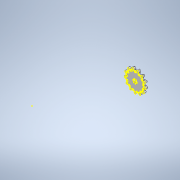
# Autodesk Inventor part: ｍ2歯数13ギア6切削実験甲
Saved by Autodesk Inventor 2020.2 (Build 242310000, 310)
## iProperties
Created: 2020-02-20
Part Number: ｍ2歯数13ギア6切削実験甲
Material: 一般
Document SubType Name: Modeling
Designer: aoyam
Density: 1 g/cm^3
Appearance: 既定
Author: aoyam
Autodesk Inventor part; units mm, degrees
ref_plane "YZ Plane" through (0, 0, 0) normal (1, 0, 0) x (0, 1, 0)
ref_plane "XZ Plane" through (0, 0, 0) normal (0, 1, 0) x (-1, 0, 0)
ref_plane "XY Plane" through (0, 0, 0) normal (0, 0, 1) x (1, 0, 0)
sketch "スケッチ1" plane through (0, 0, 0) normal (0, 0, 1) x (1, 0, 0)
  arc A0 (142.3096, 112.4021) -> (142.2446, 112.1427) centre (143.6618, 111.9254) ccw
  arc A1 (142.6961, 113.2166) -> (142.3096, 112.4021) centre (146.0761, 111.114) ccw
  arc A2 (143.9239, 114.698) -> (142.6961, 113.2166) centre (148.6702, 109.5145) ccw
  arc A3 (139.6615, 112.1427) -> (139.5965, 112.4021) centre (138.2443, 111.9254) ccw
  arc A4 (139.5965, 112.4021) -> (139.21, 113.2166) centre (135.83, 111.114) ccw
  arc A5 (139.21, 113.2166) -> (137.9821, 114.698) centre (133.2359, 109.5145) ccw
  arc A6 (142.0632, 110.4363) -> (139.8429, 110.4363) centre (140.953, 99.9952) ccw
  arc A7 (137.9821, 114.698) -> (136.7509, 114.3945) centre (140.953, 99.9952) ccw
  line L0 (142.0632, 110.4363) -> (142.2446, 112.1427)
  line L1 (139.8429, 110.4363) -> (139.6615, 112.1427)
  arc A8 (136.3884, 111.6113) -> (136.4514, 111.3515) centre (137.8072, 111.8177) ccw
  line L2 (137.0838, 109.7563) -> (136.4514, 111.3515)
  arc A9 (136.3521, 112.5122) -> (136.3884, 111.6113) centre (140.3221, 112.2212) ccw
  arc A10 (136.7509, 114.3945) -> (136.3521, 112.5122) centre (143.3624, 112.0105) ccw
  arc A11 (137.0838, 109.7563) -> (135.1178, 108.7244) centre (140.953, 99.9952) ccw
  line L3 (135.1178, 108.7244) -> (134.1642, 110.1511)
  arc A12 (134.1642, 110.1511) -> (133.9861, 110.3505) centre (133.0103, 109.3001) ccw
  arc A13 (133.9861, 110.3505) -> (133.2653, 110.8922) centre (131.2496, 107.4596) ccw
  arc A14 (133.2653, 110.8922) -> (131.4897, 111.6333) centre (129.696, 104.8378) ccw
  arc A15 (131.4897, 111.6333) -> (130.5405, 110.7923) centre (140.953, 99.9952) ccw
  arc A16 (131.513, 108.1595) -> (131.6895, 107.9587) centre (132.6734, 109.0016) ccw
  line L4 (132.9908, 106.84) -> (131.6895, 107.9587)
  arc A17 (131.0621, 108.9403) -> (131.513, 108.1595) centre (134.7127, 110.5276) ccw
  arc A18 (130.5405, 110.7923) -> (131.0621, 108.9403) centre (137.5026, 111.7539) ccw
  arc A19 (132.9908, 106.84) -> (131.7295, 105.0128) centre (140.953, 99.9952) ccw
  line L5 (131.7295, 105.0128) -> (130.2221, 105.8328)
  arc A20 (130.2221, 105.8328) -> (129.9718, 105.9267) centre (129.5959, 104.5431) ccw
  arc A21 (129.9718, 105.9267) -> (129.0818, 106.0713) centre (128.8922, 102.0952) ccw
  arc A22 (129.0818, 106.0713) -> (127.1652, 105.9023) centre (128.7349, 99.0517) ccw
  arc A23 (127.1652, 105.9023) -> (126.7155, 104.7166) centre (140.953, 99.9952) ccw
  arc A24 (128.8001, 102.8373) -> (129.0498, 102.7416) centre (129.4363, 104.1222) ccw
  line L6 (130.7218, 102.3558) -> (129.0498, 102.7416)
  arc A25 (128.0381, 103.3192) -> (128.8001, 102.8373) centre (130.5328, 106.4211) ccw
  arc A26 (126.7155, 104.7166) -> (128.0381, 103.3192) centre (132.4333, 108.8035) ccw
  arc A27 (130.7218, 102.3558) -> (130.4542, 100.1517) centre (140.953, 99.9952) ccw
  line L7 (130.4542, 100.1517) -> (128.7384, 100.1772)
  arc A28 (128.7384, 100.1772) -> (128.4731, 100.144) centre (128.7832, 98.7442) ccw
  arc A29 (128.4731, 100.144) -> (127.6179, 99.8585) centre (129.2978, 96.2497) ccw
  arc A30 (127.6179, 99.8585) -> (125.9993, 98.8182) centre (130.5729, 93.4817) ccw
  arc A31 (125.9993, 98.8182) -> (126.1521, 97.5593) centre (140.953, 99.9952) ccw
  arc A32 (128.8714, 96.864) -> (129.1369, 96.8952) centre (128.8375, 98.2974) ccw
  line L8 (130.7967, 97.3307) -> (129.1369, 96.8952)
  arc A33 (127.9727, 96.9365) -> (128.8714, 96.864) centre (128.7401, 100.8426) ccw
  arc A34 (126.1521, 97.5593) -> (127.9727, 96.9365) centre (129.3158, 103.8352) ccw
  arc A35 (130.7967, 97.3307) -> (131.5841, 95.2547) centre (140.953, 99.9952) ccw
  line L9 (131.5841, 95.2547) -> (130.0529, 94.48)
  arc A36 (130.0529, 94.48) -> (129.8334, 94.3272) centre (130.7586, 93.2319) ccw
  arc A37 (129.8334, 94.3272) -> (129.2089, 93.677) centre (132.3734, 91.2622) ccw
  arc A38 (129.2089, 93.677) -> (128.2591, 92.0036) centre (134.7888, 89.4039) ccw
  arc A39 (128.2591, 92.0036) -> (128.9795, 90.96) centre (140.953, 99.9952) ccw
  arc A40 (131.7104, 91.608) -> (131.931, 91.7591) centre (131.0143, 92.8615) ccw
  line L10 (133.1983, 92.916) -> (131.931, 91.7591)
  arc A41 (130.8809, 91.2546) -> (131.7104, 91.608) centre (129.7452, 95.0699) ccw
  arc A42 (128.9795, 90.96) -> (130.8809, 91.2546) centre (128.8642, 97.9872) ccw
  arc A43 (133.1983, 92.916) -> (134.8602, 91.4437) centre (140.953, 99.9952) ccw
  line L11 (134.8602, 91.4437) -> (133.8645, 90.0461)
  arc A44 (133.8645, 90.0461) -> (133.7411, 89.8089) centre (135.0693, 89.269) ccw
  arc A45 (133.7411, 89.8089) -> (133.4903, 88.9429) centre (137.4146, 88.2754) ccw
  arc A46 (133.4903, 88.9429) -> (133.427, 87.0199) centre (140.4169, 87.7524) ccw
  arc A47 (133.427, 87.0199) -> (134.5498, 86.4305) centre (140.953, 99.9952) ccw
  arc A48 (136.6667, 88.2735) -> (136.7919, 88.5097) centre (135.4679, 89.0598) ccw
  line L12 (137.3764, 90.1231) -> (136.7919, 88.5097)
  arc A49 (136.0966, 87.575) -> (136.6667, 88.2735) centre (133.3179, 90.4255) ccw
  arc A50 (134.5498, 86.4305) -> (136.0966, 87.575) centre (131.182, 92.5993) ccw
  arc A51 (137.3764, 90.1231) -> (139.5322, 89.5917) centre (140.953, 99.9952) ccw
  line L13 (139.5322, 89.5917) -> (139.3, 87.8915)
  arc A52 (139.3, 87.8915) -> (139.301, 87.6242) centre (140.728, 87.7633) ccw
  arc A53 (139.301, 87.6242) -> (139.4813, 86.7408) centre (143.2663, 87.9734) ccw
  arc A54 (139.4813, 86.7408) -> (140.319, 85.0086) centre (146.1678, 88.9056) ccw
  arc A55 (140.319, 85.0086) -> (141.5871, 85.0086) centre (140.953, 99.9952) ccw
  arc A56 (142.6051, 87.6242) -> (142.6061, 87.8915) centre (141.1781, 87.7633) ccw
  line L14 (142.3739, 89.5917) -> (142.6061, 87.8915)
  arc A57 (142.4248, 86.7408) -> (142.6051, 87.6242) centre (138.6397, 87.9734) ccw
  arc A58 (141.5871, 85.0086) -> (142.4248, 86.7408) centre (135.7383, 88.9056) ccw
  arc A59 (142.3739, 89.5917) -> (144.5297, 90.1231) centre (140.953, 99.9952) ccw
  line L15 (144.5297, 90.1231) -> (145.1142, 88.5097)
  arc A60 (145.1142, 88.5097) -> (145.2393, 88.2735) centre (146.4382, 89.0598) ccw
  arc A61 (145.2393, 88.2735) -> (145.8095, 87.575) centre (148.5882, 90.4255) ccw
  arc A62 (145.8095, 87.575) -> (147.3562, 86.4305) centre (150.7241, 92.5993) ccw
  arc A63 (147.3562, 86.4305) -> (148.4791, 87.0199) centre (140.953, 99.9952) ccw
  arc A64 (148.1649, 89.8089) -> (148.0416, 90.0461) centre (146.8367, 89.269) ccw
  line L16 (147.0458, 91.4437) -> (148.0416, 90.0461)
  arc A65 (148.4158, 88.9429) -> (148.1649, 89.8089) centre (144.4915, 88.2754) ccw
  arc A66 (148.4791, 87.0199) -> (148.4158, 88.9429) centre (141.4892, 87.7524) ccw
  arc A67 (147.0458, 91.4437) -> (148.7078, 92.916) centre (140.953, 99.9952) ccw
  line L17 (148.7078, 92.916) -> (149.9751, 91.7591)
  arc A68 (149.9751, 91.7591) -> (150.1957, 91.608) centre (150.8918, 92.8615) ccw
  arc A69 (150.1957, 91.608) -> (151.0252, 91.2546) centre (152.1608, 95.0699) ccw
  arc A70 (151.0252, 91.2546) -> (152.9266, 90.96) centre (153.0419, 97.9872) ccw
  arc A71 (152.9266, 90.96) -> (153.6469, 92.0036) centre (140.953, 99.9952) ccw
  arc A72 (152.0726, 94.3272) -> (151.8532, 94.48) centre (151.1475, 93.2319) ccw
  line L18 (150.322, 95.2547) -> (151.8532, 94.48)
  arc A73 (152.6972, 93.677) -> (152.0726, 94.3272) centre (149.5326, 91.2622) ccw
  arc A74 (153.6469, 92.0036) -> (152.6972, 93.677) centre (147.1172, 89.4039) ccw
  arc A75 (150.322, 95.2547) -> (151.1093, 97.3307) centre (140.953, 99.9952) ccw
  line L19 (151.1093, 97.3307) -> (152.7692, 96.8952)
  arc A76 (152.7692, 96.8952) -> (153.0347, 96.864) centre (153.0686, 98.2974) ccw
  arc A77 (153.0347, 96.864) -> (153.9334, 96.9365) centre (153.166, 100.8426) ccw
  arc A78 (153.9334, 96.9365) -> (155.7539, 97.5593) centre (152.5903, 103.8352) ccw
  arc A79 (155.7539, 97.5593) -> (155.9068, 98.8182) centre (140.953, 99.9952) ccw
  arc A80 (153.433, 100.144) -> (153.1677, 100.1772) centre (153.1228, 98.7442) ccw
  line L20 (151.4519, 100.1517) -> (153.1677, 100.1772)
  arc A81 (154.2882, 99.8585) -> (153.433, 100.144) centre (152.6083, 96.2497) ccw
  arc A82 (155.9068, 98.8182) -> (154.2882, 99.8585) centre (151.3332, 93.4817) ccw
  arc A83 (151.4519, 100.1517) -> (151.1842, 102.3558) centre (140.953, 99.9952) ccw
  line L21 (151.1842, 102.3558) -> (152.8563, 102.7416)
  arc A84 (152.8563, 102.7416) -> (153.1059, 102.8373) centre (152.4698, 104.1222) ccw
  arc A85 (153.1059, 102.8373) -> (153.868, 103.3192) centre (151.3732, 106.4211) ccw
  arc A86 (153.868, 103.3192) -> (155.1906, 104.7166) centre (149.4728, 108.8035) ccw
  arc A87 (155.1906, 104.7166) -> (154.7409, 105.9023) centre (140.953, 99.9952) ccw
  arc A88 (151.9343, 105.9267) -> (151.684, 105.8328) centre (152.3102, 104.5431) ccw
  line L22 (150.1766, 105.0128) -> (151.684, 105.8328)
  arc A89 (152.8242, 106.0713) -> (151.9343, 105.9267) centre (153.0139, 102.0952) ccw
  arc A90 (154.7409, 105.9023) -> (152.8242, 106.0713) centre (153.1711, 99.0517) ccw
  arc A91 (150.1766, 105.0128) -> (148.9153, 106.84) centre (140.953, 99.9952) ccw
  line L23 (148.9153, 106.84) -> (150.2166, 107.9587)
  arc A92 (150.2166, 107.9587) -> (150.3931, 108.1595) centre (149.2327, 109.0016) ccw
  arc A93 (150.3931, 108.1595) -> (150.8439, 108.9403) centre (147.1934, 110.5276) ccw
  arc A94 (150.8439, 108.9403) -> (151.3656, 110.7923) centre (144.4035, 111.7539) ccw
  arc A95 (151.3656, 110.7923) -> (150.4164, 111.6333) centre (140.953, 99.9952) ccw
  arc A96 (147.92, 110.3505) -> (147.7419, 110.1511) centre (148.8958, 109.3001) ccw
  line L24 (146.7883, 108.7244) -> (147.7419, 110.1511)
  arc A97 (148.6407, 110.8922) -> (147.92, 110.3505) centre (150.6565, 107.4596) ccw
  arc A98 (150.4164, 111.6333) -> (148.6407, 110.8922) centre (152.2101, 104.8378) ccw
  arc A99 (146.7883, 108.7244) -> (144.8223, 109.7563) centre (140.953, 99.9952) ccw
  line L25 (144.8223, 109.7563) -> (145.4546, 111.3515)
  arc A100 (145.4546, 111.3515) -> (145.5176, 111.6113) centre (144.0988, 111.8177) ccw
  arc A101 (145.5176, 111.6113) -> (145.554, 112.5122) centre (141.5839, 112.2212) ccw
  arc A102 (145.554, 112.5122) -> (145.1552, 114.3945) centre (138.5437, 112.0105) ccw
  arc A103 (145.1552, 114.3945) -> (143.9239, 114.698) centre (140.953, 99.9952) ccw
  circle A104 centre (140.953, 99.9952) radius 10.5 construction
  circle A105 centre (140.953, 99.9952) radius 15 construction
  line L26 (140.7262, 102.7971) -> (141.8821, 102.6483)
  line L27 (143.2661, 101.5926) -> (143.7152, 100.5172)
  line L28 (143.493, 98.7907) -> (142.7862, 97.8641)
  line L29 (141.1799, 97.1933) -> (140.024, 97.3421)
  line L30 (138.64, 98.3978) -> (138.1909, 99.4732)
  line L31 (138.4131, 101.1996) -> (139.1199, 102.1263)
  arc A106 (140.7262, 102.7971) -> (139.1199, 102.1263) centre (140.1167, 101.998) ccw
  arc A107 (138.4131, 101.1996) -> (138.1909, 99.4732) centre (138.8004, 100.2723) ccw
  arc A108 (138.64, 98.3978) -> (140.024, 97.3421) centre (139.6367, 98.2694) ccw
  arc A109 (141.1799, 97.1933) -> (142.7862, 97.8641) centre (141.7894, 97.9924) ccw
  arc A110 (143.493, 98.7907) -> (143.7152, 100.5172) centre (143.1057, 99.7181) ccw
  arc A111 (143.2661, 101.5926) -> (141.8821, 102.6483) centre (142.2693, 101.7209) ccw
  point P0 (0, 0)
  point P1 (140.953, 116.9952)
  point P2 (133.0527, 115.0479)
  point P3 (126.9623, 109.6523)
  point P4 (124.077, 102.0443)
  point P5 (125.0578, 93.9669)
  point P6 (129.6799, 87.2705)
  point P7 (136.8847, 83.4892)
  point P8 (145.0214, 83.4892)
  point P9 (152.2261, 87.2705)
  point P10 (156.8483, 93.9669)
  point P11 (157.8291, 102.0443)
  point P12 (154.9438, 109.6523)
  point P13 (148.8533, 115.0479)
  point P14 (139.7294, 102.9254)
  point P15 (137.8036, 100.4006)
  point P16 (139.0272, 97.4704)
  point P17 (142.1767, 97.065)
  point P18 (144.1025, 99.5898)
  point P19 (142.8788, 102.52)
  point P20 (145.2393, 88.2735)
  point P21 (145.8095, 87.575)
  point P22 (147.3562, 86.4305)
  point P23 (148.4791, 87.0199)
  point P24 (148.4158, 88.9429)
  point P25 (148.0416, 90.0461)
  point P26 (147.0458, 91.4437)
  point P27 (148.7078, 92.916)
  point P28 (150.1957, 91.608)
  point P29 (151.0252, 91.2546)
  point P30 (152.9266, 90.96)
  point P31 (153.6469, 92.0036)
  point P32 (152.6972, 93.677)
  point P33 (152.0726, 94.3272)
  point P34 (153.0347, 96.864)
  point P35 (153.9334, 96.9365)
  point P36 (155.7539, 97.5593)
  point P37 (155.9068, 98.8182)
  point P38 (154.2882, 99.8585)
  point P39 (153.433, 100.144)
  point P40 (153.1677, 100.1772)
  point P41 (151.4519, 100.1517)
  point P42 (153.1059, 102.8373)
  point P43 (153.868, 103.3192)
  point P44 (155.1906, 104.7166)
  point P45 (154.7409, 105.9023)
  point P46 (152.8242, 106.0713)
  point P47 (151.9343, 105.9267)
  point P48 (150.2166, 107.9587)
  point P49 (150.3931, 108.1595)
  point P50 (151.3656, 110.7923)
  point P51 (150.4164, 111.6333)
  point P52 (148.6407, 110.8922)
  point P53 (147.7419, 110.1511)
  point P54 (145.4546, 111.3515)
  point P55 (145.5176, 111.6113)
  point P56 (145.554, 112.5122)
  point P57 (145.1552, 114.3945)
  point P58 (143.9239, 114.698)
  point P59 (142.6961, 113.2166)
  point P60 (142.2446, 112.1427)
  point P61 (139.6615, 112.1427)
  point P62 (139.5965, 112.4021)
  point P63 (139.21, 113.2166)
  point P64 (136.3884, 111.6113)
  point P65 (137.0838, 109.7563)
  point P66 (135.1178, 108.7244)
  point P67 (133.9861, 110.3505)
  point P68 (133.2653, 110.8922)
  point P69 (131.513, 108.1595)
  point P70 (130.2221, 105.8328)
  point P71 (129.0818, 106.0713)
  point P72 (127.1652, 105.9023)
  point P73 (126.7155, 104.7166)
  point P74 (128.8001, 102.8373)
  point P75 (127.6179, 99.8585)
  point P76 (126.1521, 97.5593)
  point P77 (127.9727, 96.9365)
  point P78 (128.8714, 96.864)
  point P79 (129.8334, 94.3272)
  point P80 (129.2089, 93.677)
  point P81 (128.2591, 92.0036)
  point P82 (128.9795, 90.96)
  point P83 (131.7104, 91.608)
  point P84 (133.1983, 92.916)
  point P85 (133.7411, 89.8089)
  point P86 (133.4903, 88.9429)
  point P87 (134.5498, 86.4305)
  point P88 (136.0966, 87.575)
  point P89 (136.6667, 88.2735)
  point P90 (136.7919, 88.5097)
  point P91 (137.3764, 90.1231)
  point P92 (139.301, 87.6242)
  point P93 (139.4813, 86.7408)
  point P94 (140.319, 85.0086)
  point P95 (142.4248, 86.7408)
  dimension "d4" = 360
  dimension "d10" = 5.5
  dimension "d11" = 2.01
  dimension "d14" = 360
  dimension "d18" = 30
  constraints: 226 point on circle, 112 centre point, 64 end point, 4 coincident, 1 concentric, 537 other
  measures "d10" distance between parallel lines of L30 L27
  measures "d11" diameter of A106
  measures "d18" diameter of A105
extrude "押し出し1" add sketch "スケッチ1" along normal blind 3
sketch "スケッチ2" plane through (0, 0, 3) normal (0, 0, 1) x (1, 0, 0)
  arc A0 (148.4791, 87.0199) -> (148.4158, 88.9429) centre (141.4892, 87.7524) ccw projected
  arc A1 (148.4158, 88.9429) -> (148.1649, 89.8089) centre (144.4915, 88.2754) ccw projected
  arc A2 (148.1649, 89.8089) -> (148.0416, 90.0461) centre (146.8367, 89.269) ccw projected
  line L0 (148.0416, 90.0461) -> (147.0458, 91.4437) projected
  arc A3 (147.0458, 91.4437) -> (148.7078, 92.916) centre (140.953, 99.9952) ccw projected
  line L1 (148.7078, 92.916) -> (149.9751, 91.7591) projected
  arc A4 (149.9751, 91.7591) -> (150.1957, 91.608) centre (150.8918, 92.8615) ccw projected
  arc A5 (150.1957, 91.608) -> (151.0252, 91.2546) centre (152.1608, 95.0699) ccw projected
  arc A6 (151.0252, 91.2546) -> (152.9266, 90.96) centre (153.0419, 97.9872) ccw projected
  arc A7 (152.9266, 90.96) -> (153.6469, 92.0036) centre (140.953, 99.9952) ccw projected
  arc A8 (153.6469, 92.0036) -> (152.6972, 93.677) centre (147.1172, 89.4039) ccw projected
  arc A9 (152.6972, 93.677) -> (152.0726, 94.3272) centre (149.5326, 91.2622) ccw projected
  arc A10 (152.0726, 94.3272) -> (151.8532, 94.48) centre (151.1475, 93.2319) ccw projected
  line L2 (151.8532, 94.48) -> (150.322, 95.2547) projected
  arc A11 (150.322, 95.2547) -> (151.1093, 97.3307) centre (140.953, 99.9952) ccw projected
  line L3 (151.1093, 97.3307) -> (152.7692, 96.8952) projected
  arc A12 (152.7692, 96.8952) -> (153.0347, 96.864) centre (153.0686, 98.2974) ccw projected
  arc A13 (153.0347, 96.864) -> (153.9334, 96.9365) centre (153.166, 100.8426) ccw projected
  arc A14 (153.9334, 96.9365) -> (155.7539, 97.5593) centre (152.5903, 103.8352) ccw projected
  arc A15 (155.7539, 97.5593) -> (155.9068, 98.8182) centre (140.953, 99.9952) ccw projected
  arc A16 (155.9068, 98.8182) -> (154.2882, 99.8585) centre (151.3332, 93.4817) ccw projected
  arc A17 (154.2882, 99.8585) -> (153.433, 100.144) centre (152.6083, 96.2497) ccw projected
  arc A18 (153.433, 100.144) -> (153.1677, 100.1772) centre (153.1228, 98.7442) ccw projected
  line L4 (153.1677, 100.1772) -> (151.4519, 100.1517) projected
  arc A19 (151.4519, 100.1517) -> (151.1842, 102.3558) centre (140.953, 99.9952) ccw projected
  line L5 (151.1842, 102.3558) -> (152.8563, 102.7416) projected
  arc A20 (152.8563, 102.7416) -> (153.1059, 102.8373) centre (152.4698, 104.1222) ccw projected
  arc A21 (153.1059, 102.8373) -> (153.868, 103.3192) centre (151.3732, 106.4211) ccw projected
  arc A22 (153.868, 103.3192) -> (155.1906, 104.7166) centre (149.4728, 108.8035) ccw projected
  arc A23 (155.1906, 104.7166) -> (154.7409, 105.9023) centre (140.953, 99.9952) ccw projected
  arc A24 (154.7409, 105.9023) -> (152.8242, 106.0713) centre (153.1711, 99.0517) ccw projected
  arc A25 (152.8242, 106.0713) -> (151.9343, 105.9267) centre (153.0139, 102.0952) ccw projected
  arc A26 (151.9343, 105.9267) -> (151.684, 105.8328) centre (152.3102, 104.5431) ccw projected
  line L6 (151.684, 105.8328) -> (150.1766, 105.0128) projected
  arc A27 (150.1766, 105.0128) -> (148.9153, 106.84) centre (140.953, 99.9952) ccw projected
  line L7 (148.9153, 106.84) -> (150.2166, 107.9587) projected
  arc A28 (150.2166, 107.9587) -> (150.3931, 108.1595) centre (149.2327, 109.0016) ccw projected
  arc A29 (150.3931, 108.1595) -> (150.8439, 108.9403) centre (147.1934, 110.5276) ccw projected
  arc A30 (150.8439, 108.9403) -> (151.3656, 110.7923) centre (144.4035, 111.7539) ccw projected
  arc A31 (151.3656, 110.7923) -> (150.4164, 111.6333) centre (140.953, 99.9952) ccw projected
  arc A32 (150.4164, 111.6333) -> (148.6407, 110.8922) centre (152.2101, 104.8378) ccw projected
  arc A33 (148.6407, 110.8922) -> (147.92, 110.3505) centre (150.6565, 107.4596) ccw projected
  arc A34 (147.92, 110.3505) -> (147.7419, 110.1511) centre (148.8958, 109.3001) ccw projected
  line L8 (147.7419, 110.1511) -> (146.7883, 108.7244) projected
  arc A35 (146.7883, 108.7244) -> (144.8223, 109.7563) centre (140.953, 99.9952) ccw projected
  line L9 (144.8223, 109.7563) -> (145.4546, 111.3515) projected
  arc A36 (145.4546, 111.3515) -> (145.5176, 111.6113) centre (144.0988, 111.8177) ccw projected
  arc A37 (145.5176, 111.6113) -> (145.554, 112.5122) centre (141.5839, 112.2212) ccw projected
  arc A38 (145.554, 112.5122) -> (145.1552, 114.3945) centre (138.5437, 112.0105) ccw projected
  arc A39 (145.1552, 114.3945) -> (143.9239, 114.698) centre (140.953, 99.9952) ccw projected
  arc A40 (143.9239, 114.698) -> (142.6961, 113.2166) centre (148.6702, 109.5145) ccw projected
  arc A41 (142.6961, 113.2166) -> (142.3096, 112.4021) centre (146.0761, 111.114) ccw projected
  arc A42 (142.3096, 112.4021) -> (142.2446, 112.1427) centre (143.6618, 111.9254) ccw projected
  line L10 (142.2446, 112.1427) -> (142.0632, 110.4363) projected
  arc A43 (142.0632, 110.4363) -> (139.8429, 110.4363) centre (140.953, 99.9952) ccw projected
  line L11 (139.8429, 110.4363) -> (139.6615, 112.1427) projected
  arc A44 (139.6615, 112.1427) -> (139.5965, 112.4021) centre (138.2443, 111.9254) ccw projected
  arc A45 (139.5965, 112.4021) -> (139.21, 113.2166) centre (135.83, 111.114) ccw projected
  arc A46 (139.21, 113.2166) -> (137.9821, 114.698) centre (133.2359, 109.5145) ccw projected
  arc A47 (137.9821, 114.698) -> (136.7509, 114.3945) centre (140.953, 99.9952) ccw projected
  arc A48 (136.7509, 114.3945) -> (136.3521, 112.5122) centre (143.3624, 112.0105) ccw projected
  arc A49 (136.3521, 112.5122) -> (136.3884, 111.6113) centre (140.3221, 112.2212) ccw projected
  arc A50 (136.3884, 111.6113) -> (136.4514, 111.3515) centre (137.8072, 111.8177) ccw projected
  line L12 (136.4514, 111.3515) -> (137.0838, 109.7563) projected
  arc A51 (137.0838, 109.7563) -> (135.1178, 108.7244) centre (140.953, 99.9952) ccw projected
  line L13 (135.1178, 108.7244) -> (134.1642, 110.1511) projected
  arc A52 (134.1642, 110.1511) -> (133.9861, 110.3505) centre (133.0103, 109.3001) ccw projected
  arc A53 (133.9861, 110.3505) -> (133.2653, 110.8922) centre (131.2496, 107.4596) ccw projected
  arc A54 (133.2653, 110.8922) -> (131.4897, 111.6333) centre (129.696, 104.8378) ccw projected
  arc A55 (131.4897, 111.6333) -> (130.5405, 110.7923) centre (140.953, 99.9952) ccw projected
  arc A56 (130.5405, 110.7923) -> (131.0621, 108.9403) centre (137.5026, 111.7539) ccw projected
  arc A57 (131.0621, 108.9403) -> (131.513, 108.1595) centre (134.7127, 110.5276) ccw projected
  arc A58 (131.513, 108.1595) -> (131.6895, 107.9587) centre (132.6734, 109.0016) ccw projected
  line L14 (131.6895, 107.9587) -> (132.9908, 106.84) projected
  arc A59 (132.9908, 106.84) -> (131.7295, 105.0128) centre (140.953, 99.9952) ccw projected
  line L15 (131.7295, 105.0128) -> (130.2221, 105.8328) projected
  arc A60 (130.2221, 105.8328) -> (129.9718, 105.9267) centre (129.5959, 104.5431) ccw projected
  arc A61 (129.9718, 105.9267) -> (129.0818, 106.0713) centre (128.8922, 102.0952) ccw projected
  arc A62 (129.0818, 106.0713) -> (127.1652, 105.9023) centre (128.7349, 99.0517) ccw projected
  arc A63 (127.1652, 105.9023) -> (126.7155, 104.7166) centre (140.953, 99.9952) ccw projected
  arc A64 (126.7155, 104.7166) -> (128.0381, 103.3192) centre (132.4333, 108.8035) ccw projected
  arc A65 (128.0381, 103.3192) -> (128.8001, 102.8373) centre (130.5328, 106.4211) ccw projected
  arc A66 (128.8001, 102.8373) -> (129.0498, 102.7416) centre (129.4363, 104.1222) ccw projected
  line L16 (129.0498, 102.7416) -> (130.7218, 102.3558) projected
  arc A67 (130.7218, 102.3558) -> (130.4542, 100.1517) centre (140.953, 99.9952) ccw projected
  line L17 (130.4542, 100.1517) -> (128.7384, 100.1772) projected
  arc A68 (128.7384, 100.1772) -> (128.4731, 100.144) centre (128.7832, 98.7442) ccw projected
  arc A69 (128.4731, 100.144) -> (127.6179, 99.8585) centre (129.2978, 96.2497) ccw projected
  arc A70 (127.6179, 99.8585) -> (125.9993, 98.8182) centre (130.5729, 93.4817) ccw projected
  arc A71 (125.9993, 98.8182) -> (126.1521, 97.5593) centre (140.953, 99.9952) ccw projected
  arc A72 (126.1521, 97.5593) -> (127.9727, 96.9365) centre (129.3158, 103.8352) ccw projected
  arc A73 (127.9727, 96.9365) -> (128.8714, 96.864) centre (128.7401, 100.8426) ccw projected
  arc A74 (128.8714, 96.864) -> (129.1369, 96.8952) centre (128.8375, 98.2974) ccw projected
  line L18 (129.1369, 96.8952) -> (130.7967, 97.3307) projected
  arc A75 (130.7967, 97.3307) -> (131.5841, 95.2547) centre (140.953, 99.9952) ccw projected
  line L19 (131.5841, 95.2547) -> (130.0529, 94.48) projected
  arc A76 (130.0529, 94.48) -> (129.8334, 94.3272) centre (130.7586, 93.2319) ccw projected
  arc A77 (129.8334, 94.3272) -> (129.2089, 93.677) centre (132.3734, 91.2622) ccw projected
  arc A78 (129.2089, 93.677) -> (128.2591, 92.0036) centre (134.7888, 89.4039) ccw projected
  arc A79 (128.2591, 92.0036) -> (128.9795, 90.96) centre (140.953, 99.9952) ccw projected
  arc A80 (128.9795, 90.96) -> (130.8809, 91.2546) centre (128.8642, 97.9872) ccw projected
  arc A81 (130.8809, 91.2546) -> (131.7104, 91.608) centre (129.7452, 95.0699) ccw projected
  arc A82 (131.7104, 91.608) -> (131.931, 91.7591) centre (131.0143, 92.8615) ccw projected
  line L20 (131.931, 91.7591) -> (133.1983, 92.916) projected
  arc A83 (133.1983, 92.916) -> (134.8602, 91.4437) centre (140.953, 99.9952) ccw projected
  line L21 (134.8602, 91.4437) -> (133.8645, 90.0461) projected
  arc A84 (133.8645, 90.0461) -> (133.7411, 89.8089) centre (135.0693, 89.269) ccw projected
  arc A85 (133.7411, 89.8089) -> (133.4903, 88.9429) centre (137.4146, 88.2754) ccw projected
  arc A86 (133.4903, 88.9429) -> (133.427, 87.0199) centre (140.4169, 87.7524) ccw projected
  arc A87 (133.427, 87.0199) -> (134.5498, 86.4305) centre (140.953, 99.9952) ccw projected
  arc A88 (134.5498, 86.4305) -> (136.0966, 87.575) centre (131.182, 92.5993) ccw projected
  arc A89 (136.0966, 87.575) -> (136.6667, 88.2735) centre (133.3179, 90.4255) ccw projected
  arc A90 (136.6667, 88.2735) -> (136.7919, 88.5097) centre (135.4679, 89.0598) ccw projected
  line L22 (136.7919, 88.5097) -> (137.3764, 90.1231) projected
  arc A91 (137.3764, 90.1231) -> (139.5322, 89.5917) centre (140.953, 99.9952) ccw projected
  line L23 (139.5322, 89.5917) -> (139.3, 87.8915) projected
  arc A92 (139.3, 87.8915) -> (139.301, 87.6242) centre (140.728, 87.7633) ccw projected
  arc A93 (139.301, 87.6242) -> (139.4813, 86.7408) centre (143.2663, 87.9734) ccw projected
  arc A94 (139.4813, 86.7408) -> (140.319, 85.0086) centre (146.1678, 88.9056) ccw projected
  arc A95 (140.319, 85.0086) -> (141.5871, 85.0086) centre (140.953, 99.9952) ccw projected
  arc A96 (141.5871, 85.0086) -> (142.4248, 86.7408) centre (135.7383, 88.9056) ccw projected
  arc A97 (142.4248, 86.7408) -> (142.6051, 87.6242) centre (138.6397, 87.9734) ccw projected
  arc A98 (142.6051, 87.6242) -> (142.6061, 87.8915) centre (141.1781, 87.7633) ccw projected
  line L24 (142.6061, 87.8915) -> (142.3739, 89.5917) projected
  arc A99 (142.3739, 89.5917) -> (144.5297, 90.1231) centre (140.953, 99.9952) ccw projected
  line L25 (144.5297, 90.1231) -> (145.1142, 88.5097) projected
  arc A100 (145.1142, 88.5097) -> (145.2393, 88.2735) centre (146.4382, 89.0598) ccw projected
  arc A101 (145.2393, 88.2735) -> (145.8095, 87.575) centre (148.5882, 90.4255) ccw projected
  arc A102 (145.8095, 87.575) -> (147.3562, 86.4305) centre (150.7241, 92.5993) ccw projected
  arc A103 (147.3562, 86.4305) -> (148.4791, 87.0199) centre (140.953, 99.9952) ccw projected
  line L26 (138.4131, 101.1996) -> (139.1199, 102.1263) projected
  arc A104 (140.7262, 102.7971) -> (139.1199, 102.1263) centre (140.1167, 101.998) ccw projected
  line L27 (140.7262, 102.7971) -> (141.8821, 102.6483) projected
  arc A105 (143.2661, 101.5926) -> (141.8821, 102.6483) centre (142.2693, 101.7209) ccw projected
  line L28 (143.2661, 101.5926) -> (143.7152, 100.5172) projected
  arc A106 (143.493, 98.7907) -> (143.7152, 100.5172) centre (143.1057, 99.7181) ccw projected
  line L29 (143.493, 98.7907) -> (142.7862, 97.8641) projected
  arc A107 (141.1799, 97.1933) -> (142.7862, 97.8641) centre (141.7894, 97.9924) ccw projected
  line L30 (141.1799, 97.1933) -> (140.024, 97.3421) projected
  arc A108 (138.64, 98.3978) -> (140.024, 97.3421) centre (139.6367, 98.2694) ccw projected
  line L31 (138.64, 98.3978) -> (138.1909, 99.4732) projected
  arc A109 (138.4131, 101.1996) -> (138.1909, 99.4732) centre (138.8004, 100.2723) ccw projected
  point P0 (0, 0)
